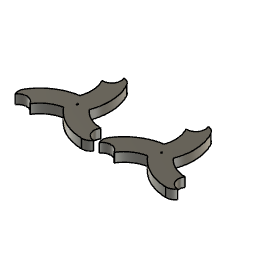
wheel v1 (Autodesk Fusion 360 design; units mm, degrees)
Autodesk Fusion 360 part; units mm, degrees
note: some values were not read from the file. Set by a fixed rule: which sketch regions a step uses.
sketch "스케치1" plane through (0, 0, 0) normal (0, 0, 1) x (1, 0, 0)
  arc A0 (-0.9923, 8.7365) -> (-0.9923, -1.7365) centre (2, 3.5) ccw
  arc A1 (0.9923, 5.2635) -> (-0.9923, 8.7365) centre (0, 7) ccw
  arc A2 (0.9923, 5.2635) -> (0.9923, 1.7365) centre (2, 3.5) ccw
  arc A3 (-0.9923, -1.7365) -> (0.9923, 1.7365) centre (0, 0) ccw
  arc A4 (0, 7) -> (0, 0) centre (2, 3.5) ccw construction
  arc A5 (-7.0699, -5.2276) -> (2, 0.0089) centre (-4.0311, -0.0179) ccw
  arc A6 (-5.0545, -1.7724) -> (-7.0699, -5.2276) centre (-6.0622, -3.5) ccw
  arc A7 (-6.0622, -3.5) -> (0, 0) centre (-4.0311, -0.0179) ccw construction
  arc A8 (-5.0545, -1.7724) -> (-2, -0.0089) centre (-4.0311, -0.0179) ccw
  arc A9 (2, 0.0089) -> (-2, -0.0089) centre (0, 0) ccw
  arc A10 (8.0622, -3.5089) -> (-1.0077, 1.7276) centre (2.0311, -3.4821) ccw
  arc A11 (4.0622, -3.4911) -> (8.0622, -3.5089) centre (6.0622, -3.5) ccw
  arc A12 (6.0622, -3.5) -> (0, 0) centre (2.0311, -3.4821) ccw construction
  arc A13 (4.0622, -3.4911) -> (1.0077, -1.7276) centre (2.0311, -3.4821) ccw
  arc A14 (-1.0077, 1.7276) -> (1.0077, -1.7276) centre (0, 0) ccw
  dimension "d7" = 4
  dimension "d9" = 360
  constraint tangent A0 A1
  constraint tangent A1 A2
  constraint tangent A2 A3
  constraint tangent A0 A3
  constraint coincident A3.centre A4.end
  measures "d7" diameter of A3
sketch "스케치2" plane through (0, 0, 0) normal (0, 0, 1) x (1, 0, 0)
  arc A0 (18.3127, 8.0738) -> (18.3127, -1.0738) centre (25.5, 3.5) ccw
  arc A1 (21.6873, 5.9262) -> (18.3127, 8.0738) centre (20, 7) ccw
  arc A2 (21.6873, 5.9262) -> (21.6873, 1.0738) centre (25.5, 3.5) ccw
  arc A3 (18.3127, -1.0738) -> (21.6873, 1.0738) centre (20, 0) ccw
  arc A4 (20, 7) -> (20, 0) centre (25.5, 3.5) ccw construction
  arc A5 (21.7736, -0.9244) -> (18.2264, 0.9244) centre (20, 0) ccw
  arc A6 (14.0241, -1.5019) -> (18.2264, 0.9244) centre (14.2189, 3.0131) ccw
  arc A7 (13.8516, -5.4981) -> (21.7736, -0.9244) centre (14.2189, 3.0131) ccw
  arc A8 (13.9378, -3.5) -> (20, 0) centre (14.2189, 3.0131) ccw construction
  arc A9 (14.0241, -1.5019) -> (13.8516, -5.4981) centre (13.9378, -3.5) ccw
  arc A10 (19.9138, 1.9981) -> (20.0862, -1.9981) centre (20, 0) ccw
  arc A11 (24.2886, -4.4244) -> (20.0862, -1.9981) centre (20.2811, -6.5131) ccw
  arc A12 (27.8357, -2.5756) -> (19.9138, 1.9981) centre (20.2811, -6.5131) ccw
  arc A13 (26.0622, -3.5) -> (20, 0) centre (20.2811, -6.5131) ccw construction
  arc A14 (24.2886, -4.4244) -> (27.8357, -2.5756) centre (26.0622, -3.5) ccw
  arc A15 (-21.3613, 8.4652) -> (-21.3613, -1.4652) centre (-16.7482, 3.5) ccw
  arc A16 (-18.6387, 5.5348) -> (-21.3613, 8.4652) centre (-20, 7) ccw
  arc A17 (-18.6387, 5.5348) -> (-18.6387, 1.4652) centre (-16.7482, 3.5) ccw
  arc A18 (-21.3613, -1.4652) -> (-18.6387, 1.4652) centre (-20, 0) ccw
  arc A19 (-20, 7) -> (-20, 0) centre (-16.7482, 3.5) ccw construction
  arc A20 (-18.0504, -0.4463) -> (-21.9496, 0.4463) centre (-20, 0) ccw
  arc A21 (-26.6504, -5.4115) -> (-18.0504, -0.4463) centre (-24.657, 1.0661) ccw
  arc A22 (-25.4739, -1.5885) -> (-26.6504, -5.4115) centre (-26.0622, -3.5) ccw
  arc A23 (-25.4739, -1.5885) -> (-21.9496, 0.4463) centre (-24.657, 1.0661) ccw
  arc A24 (-26.0622, -3.5) -> (-20, 0) centre (-24.657, 1.0661) ccw construction
  arc A25 (-20.5883, 1.9115) -> (-19.4117, -1.9115) centre (-20, 0) ccw
  arc A26 (-11.9883, -3.0537) -> (-20.5883, 1.9115) centre (-18.5948, -4.5661) ccw
  arc A27 (-15.8874, -3.9463) -> (-11.9883, -3.0537) centre (-13.9378, -3.5) ccw
  arc A28 (-15.8874, -3.9463) -> (-19.4117, -1.9115) centre (-18.5948, -4.5661) ccw
  arc A29 (-13.9378, -3.5) -> (-20, 0) centre (-18.5948, -4.5661) ccw construction
  dimension "d12" = 4
  dimension "d14" = 360
  dimension "d15" = 7
  dimension "d16" = 4
  dimension "d18" = 360
  constraint tangent A0 A1
  constraint tangent A1 A2
  constraint tangent A2 A3
  constraint tangent A0 A3
  constraint tangent A15 A16
  constraint tangent A16 A17
  constraint tangent A17 A18
  constraint tangent A15 A18
  measures "d12" diameter of A3
  measures "d15" distance of A18.centre A16.centre
  measures "d16" diameter of A18
sketch "스케치3" plane through (0, 0, 3) normal (0, 0, 1) x (-1, 0, 0)
  arc A0 (11.9883, 3.0537) -> (19.1945, -2.1847) centre (18.5948, 4.5661) ccw
  arc A1 (18.6387, -5.5348) -> (19.1945, -2.1847) centre (16.7482, -3.5) ccw
  arc A2 (18.6387, -5.5348) -> (21.3613, -8.4652) centre (20, -7) ccw
  arc A3 (21.3613, -8.4652) -> (22.2948, 0.3948) centre (16.7482, -3.5) ccw
  arc A4 (25.4739, 1.5885) -> (22.2948, 0.3948) centre (24.657, -1.0661) ccw
  arc A5 (25.4739, 1.5885) -> (26.6504, 5.4115) centre (26.0622, 3.5) ccw
  arc A6 (26.6504, 5.4115) -> (18.5107, 1.7899) centre (24.657, -1.0661) ccw
  arc A7 (15.8874, 3.9463) -> (18.5107, 1.7899) centre (18.5948, 4.5661) ccw
  arc A8 (15.8874, 3.9463) -> (11.9883, 3.0537) centre (13.9378, 3.5) ccw
  circle A9 centre (20, 0) radius 2.5
  arc A10 (-286.7011, -14.9378) -> (-286.7011, -55.0622) centre (-268.8401, -35) ccw
  arc A11 (-286.7011, -14.9378) -> (-313.2989, 14.9378) centre (-300, 0) ccw
  arc A12 (-313.2989, 14.9378) -> (-313.2989, -84.9378) centre (-268.8401, -35) ccw
  arc A13 (-313.2989, -84.9378) -> (-286.7011, -55.0622) centre (-300, -70) ccw
  arc A14 (-300, 0) -> (-300, -70) centre (-268.8401, -35) ccw construction
  arc A15 (-306.2871, -18.9861) -> (-219.7922, 30.9517) centre (-285.269, 44.4852) ccw
  arc A16 (-293.7129, 18.9861) -> (-258.9642, 39.0483) centre (-285.269, 44.4852) ccw
  arc A17 (-300, 0) -> (-239.3782, 35) centre (-285.269, 44.4852) ccw construction
  arc A18 (-219.7922, 30.9517) -> (-258.9642, 39.0483) centre (-239.3782, 35) ccw
  arc A19 (-293.7129, 18.9861) -> (-306.2871, -18.9861) centre (-300, 0) ccw
  arc A20 (-280.414, 4.0483) -> (-366.9089, 53.9861) centre (-345.8908, -9.4852) ccw
  arc A21 (-319.586, -4.0483) -> (-354.3347, 16.0139) centre (-345.8908, -9.4852) ccw
  arc A22 (-300, 0) -> (-360.6218, 35) centre (-345.8908, -9.4852) ccw construction
  arc A23 (-366.9089, 53.9861) -> (-354.3347, 16.0139) centre (-360.6218, 35) ccw
  arc A24 (-319.586, -4.0483) -> (-280.414, 4.0483) centre (-300, 0) ccw
  dimension "d21" = 5
  dimension "d22" = 70
  dimension "d23" = 40
  dimension "d25" = 360
  constraint tangent A10 A11
  constraint tangent A11 A12
  constraint tangent A12 A13
  constraint tangent A10 A13
  measures "d21" diameter of A9
  measures "d22" distance of A13.centre A11.centre
  measures "d23" diameter of A11
sketch "스케치4" plane through (0, 0, 33) normal (0, 0, 1) x (-1, 0, 0)
  arc A0 (-284.7746, 17.629) -> (-366.9089, 53.9861) centre (-345.8908, -9.4852) ccw
  arc A1 (-366.9089, 53.9861) -> (-354.3347, 16.0139) centre (-360.6218, 35) ccw
  arc A2 (-322.8798, 4.3711) -> (-354.3347, 16.0139) centre (-345.8908, -9.4852) ccw
  arc A3 (-322.8798, 4.3711) -> (-313.2989, -84.9378) centre (-268.8401, -35) ccw
  arc A4 (-313.2989, -84.9378) -> (-286.7011, -55.0622) centre (-300, -70) ccw
  arc A5 (-292.3456, -22) -> (-286.7011, -55.0622) centre (-268.8401, -35) ccw
  arc A6 (-292.3456, -22) -> (-219.7922, 30.9517) centre (-285.269, 44.4852) ccw
  arc A7 (-219.7922, 30.9517) -> (-258.9642, 39.0483) centre (-239.3782, 35) ccw
  arc A8 (-284.7746, 17.629) -> (-258.9642, 39.0483) centre (-285.269, 44.4852) ccw
  circle A9 centre (-300, 0) radius 2.5
  line L0 (-297.5, 0) -> (-302, 0)
  line L1 (-302, -1.5) -> (-302, 1.5)
  dimension "d28" = 5
  dimension "d29" = 4.5
  constraint coincident A9 L0.start
  constraint horizontal L0
  constraint coincident A9 L1.start
  constraint coincident A9 L1.end
  constraint perpendicular L0 L1
  measures "d28" diameter of A9
  measures "d29" distance of L0.start L0.end
sketch "스케치5" plane through (0, 0, 33) normal (0, 0, 1) x (-1, 0, 0)
  line L0 (-302, -1.5) -> (-302, 1.5)
  arc A0 (-297.5, 0) -> (-302, 1.5) centre (-300, 0) ccw
  arc A1 (-302, -1.5) -> (-297.5, 0) centre (-300, 0) ccw
  arc A2 (-284.7746, 17.629) -> (-366.9089, 53.9861) centre (-345.8908, -9.4852) ccw
  arc A3 (-366.9089, 53.9861) -> (-354.3347, 16.0139) centre (-360.6218, 35) ccw
  arc A4 (-322.8798, 4.3711) -> (-354.3347, 16.0139) centre (-345.8908, -9.4852) ccw
  arc A5 (-322.8798, 4.3711) -> (-313.2989, -84.9378) centre (-268.8401, -35) ccw
  arc A6 (-313.2989, -84.9378) -> (-286.7011, -55.0622) centre (-300, -70) ccw
  arc A7 (-292.3456, -22) -> (-286.7011, -55.0622) centre (-268.8401, -35) ccw
  arc A8 (-292.3456, -22) -> (-219.7922, 30.9517) centre (-285.269, 44.4852) ccw
  arc A9 (-219.7922, 30.9517) -> (-258.9642, 39.0483) centre (-239.3782, 35) ccw
  arc A10 (-284.7746, 17.629) -> (-258.9642, 39.0483) centre (-285.269, 44.4852) ccw
  arc A11 (-572, -21) -> (-572, -99) centre (-520, -60) ccw
  arc A12 (-572, -21) -> (-628, 21) centre (-600, 0) ccw
  arc A13 (-628, 21) -> (-628, -141) centre (-520, -60) ccw
  arc A14 (-628, -141) -> (-572, -99) centre (-600, -120) ccw
  arc A15 (-600, 0) -> (-600, -120) centre (-520, -60) ccw construction
  arc A16 (-604.1865, -34.7487) -> (-463.8904, 46.2513) centre (-588.0385, 99.282) ccw
  arc A17 (-463.8904, 46.2513) -> (-528.2635, 73.7487) centre (-496.077, 60) ccw
  arc A18 (-595.8135, 34.7487) -> (-604.1865, -34.7487) centre (-600, 0) ccw
  arc A19 (-595.8135, 34.7487) -> (-528.2635, 73.7487) centre (-588.0385, 99.282) ccw
  arc A20 (-600, 0) -> (-496.077, 60) centre (-588.0385, 99.282) ccw construction
  arc A21 (-567.8135, 13.7487) -> (-708.1096, 94.7487) centre (-691.9615, -39.282) ccw
  arc A22 (-708.1096, 94.7487) -> (-699.7365, 25.2513) centre (-703.923, 60) ccw
  arc A23 (-632.1865, -13.7487) -> (-567.8135, 13.7487) centre (-600, 0) ccw
  arc A24 (-632.1865, -13.7487) -> (-699.7365, 25.2513) centre (-691.9615, -39.282) ccw
  arc A25 (-600, 0) -> (-703.923, 60) centre (-691.9615, -39.282) ccw construction
  line L1 (-600.7031, -154.9929) -> (-600.7031, 95.0071)
  line L2 (-600.7031, 95.0071) -> (-395.9953, 127.228)
  arc A26 (398.7679, -18.3054) -> (398.7679, -101.6946) centre (452.9046, -60) ccw
  arc A27 (398.7679, -18.3054) -> (351.2321, 18.3054) centre (375, 0) ccw
  arc A28 (351.2321, 18.3054) -> (351.2321, -138.3054) centre (452.9046, -60) ccw
  arc A29 (351.2321, -138.3054) -> (398.7679, -101.6946) centre (375, -120) ccw
  arc A30 (375, 0) -> (375, -120) centre (452.9046, -60) ccw construction
  arc A31 (375, 0) -> (478.923, 60) centre (388.0092, 97.4673) ccw construction
  arc A32 (378.969, 29.7363) -> (371.031, -29.7363) centre (375, 0) ccw
  arc A33 (378.969, 29.7363) -> (451.1862, 71.4309) centre (388.0092, 97.4673) ccw
  arc A34 (371.031, -29.7363) -> (506.6599, 48.5691) centre (388.0092, 97.4673) ccw
  arc A35 (506.6599, 48.5691) -> (451.1862, 71.4309) centre (478.923, 60) ccw
  arc A36 (375, 0) -> (271.077, 60) centre (284.0862, -37.4673) ccw construction
  arc A37 (347.2631, -11.4309) -> (402.7369, 11.4309) centre (375, 0) ccw
  arc A38 (347.2631, -11.4309) -> (275.0459, 30.2637) centre (284.0862, -37.4673) ccw
  arc A39 (402.7369, 11.4309) -> (267.108, 89.7363) centre (284.0862, -37.4673) ccw
  arc A40 (267.108, 89.7363) -> (275.0459, 30.2637) centre (271.077, 60) ccw
  dimension "d33" = 70
  dimension "d35" = 360
  dimension "d36" = 250
  dimension "d37" = 60
  dimension "d39" = 360
  constraint tangent A11 A12
  constraint tangent A12 A13
  constraint tangent A13 A14
  constraint tangent A11 A14
  constraint coincident A14 L1.start
  constraint vertical L1
  constraint tangent A26 A27
  constraint tangent A27 A28
  constraint tangent A28 A29
  constraint tangent A26 A29
  measures "d33" diameter of A12
  measures "d36" distance of L1.start L1.end
  measures "d37" diameter of A27
extrude "돌출5" add sketch "스케치5" along normal blind 30 contours A26 A27 A33 A34 A35 A37 A39 | A27 A32 A37 | A26 A34 A37 | A26 A28 A29 A32 A34 A37 A38 | A27 A33 A39 | A27 A28 A32 A33 A38 A39 A40 | A28 A32 A38 makes body 1
sketch "스케치6" plane through (0, 0, 63) normal (0, 0, 1) x (-1, 0, 0)
  arc A0 (393.6401, 29.368) -> (267.108, 89.7363) centre (284.0862, -37.4673) ccw
  arc A1 (267.108, 89.7363) -> (275.0459, 30.2637) centre (271.077, 60) ccw
  arc A2 (340.2465, 1.4588) -> (275.0459, 30.2637) centre (284.0862, -37.4673) ccw
  arc A3 (340.2465, 1.4588) -> (351.2321, -138.3054) centre (452.9046, -60) ccw
  arc A4 (351.2321, -138.3054) -> (398.7679, -101.6946) centre (375, -120) ccw
  arc A5 (391.1134, -30.8268) -> (398.7679, -101.6946) centre (452.9046, -60) ccw
  arc A6 (391.1134, -30.8268) -> (506.6599, 48.5691) centre (388.0092, 97.4673) ccw
  arc A7 (506.6599, 48.5691) -> (451.1862, 71.4309) centre (478.923, 60) ccw
  arc A8 (393.6401, 29.368) -> (451.1862, 71.4309) centre (388.0092, 97.4673) ccw
  circle A9 centre (375, 0) radius 2.5
  line L0 (377.5, 0) -> (373, 0)
  line L1 (373, -1.5) -> (373, 1.5)
  dimension "d42" = 5
  constraint coincident A9 L0.start
  constraint horizontal L0
  constraint coincident A9 L1.start
  constraint coincident A9 L1.end
  constraint perpendicular L0 L1
  measures "d42" diameter of A9
extrude "돌출6" cut sketch "스케치6" against normal blind 30 contours A9 L0 L1 | A9 L0 L1 bodies 1
sketch "스케치7" plane through (0, 0, 0) normal (0, 0, 1) x (1, 0, 0)
  arc A0 (-151.4706, 14.1176) -> (-151.4706, 105.8824) centre (-237.5, 60) ccw
  arc A1 (-151.4706, 14.1176) -> (-98.5294, -14.1176) centre (-125, 0) ccw
  arc A2 (-98.5294, -14.1176) -> (-98.5294, 134.1176) centre (-237.5, 60) ccw
  arc A3 (-98.5294, 134.1176) -> (-151.4706, 105.8824) centre (-125, 120) ccw
  arc A4 (-125, 0) -> (-125, 120) centre (-237.5, 60) ccw construction
  circle A5 centre (-149.8217, 136.8488) radius 30
  arc A6 (-125, 0) -> (-228.923, -60) centre (-120.7115, -127.4279) ccw construction
  arc A7 (-123.9909, -29.983) -> (-126.0091, 29.983) centre (-125, 0) ccw
  circle A8 centre (-231.1037, -89.9206) radius 30
  arc A9 (-254.3846, -44.1346) -> (-203.4615, -75.8654) centre (-228.923, -60) ccw
  arc A10 (-126.0091, 29.983) -> (-254.3846, -44.1346) centre (-120.7115, -127.4279) ccw
  arc A11 (-123.9909, -29.983) -> (-203.4615, -75.8654) centre (-120.7115, -127.4279) ccw
  arc A12 (-125, 0) -> (-21.077, -60) centre (-16.7885, 67.4279) ccw construction
  arc A13 (-99.5385, 15.8654) -> (-150.4615, -15.8654) centre (-125, 0) ccw
  circle A14 centre (5.9254, -46.9281) radius 30
  arc A15 (-22.086, -89.983) -> (-20.0679, -30.017) centre (-21.077, -60) ccw
  arc A16 (-150.4615, -15.8654) -> (-22.086, -89.983) centre (-16.7885, 67.4279) ccw
  arc A17 (-99.5385, 15.8654) -> (-20.0679, -30.017) centre (-16.7885, 67.4279) ccw
  dimension "d45" = 120
  dimension "d46" = 60
  dimension "d47" = 60
  dimension "d49" = 360
  constraint tangent A0 A1
  constraint tangent A1 A2
  constraint tangent A2 A3
  constraint tangent A0 A3
  constraint coincident A3 A5.centre
  measures "d45" distance of A3.centre A1.centre
  measures "d46" diameter of A1
  measures "d47" diameter of A5
extrude "돌출7" add sketch "스케치7" along normal blind 30 separate body contours A0 A1 A8 A9 A10 A11 A13 A16 | A1 A7 A13 | A0 A10 A13 | A0 A2 A3 A5 A7 A10 A13 A17 | A1 A11 A16 | A1 A2 A7 A11 A14 A15 A16 A17 | A2 A7 A17 makes body 2
sketch "스케치8" plane through (0, 0, 30) normal (0, 0, 1) x (-1, 0, 0)
  arc A0 (18.8963, 30.0794) -> (20.0679, 30.017) centre (21.077, 60) ccw
  arc A1 (90.4592, -3.5618) -> (20.0679, 30.017) centre (16.7885, -67.4279) ccw
  arc A2 (90.4592, -3.5618) -> (98.5294, -134.1176) centre (237.5, -60) ccw
  arc A3 (98.5294, -134.1176) -> (122.8194, -149.9206) centre (125, -120) ccw
  arc A4 (152.0023, -106.9281) -> (122.8194, -149.9206) centre (149.8217, -136.8488) ccw
  arc A5 (152.0023, -106.9281) -> (151.4706, -105.8824) centre (125, -120) ccw
  arc A6 (145.355, -28.1323) -> (151.4706, -105.8824) centre (237.5, -60) ccw
  arc A7 (145.355, -28.1323) -> (254.3846, 44.1346) centre (120.7115, 127.4279) ccw
  arc A8 (254.3846, 44.1346) -> (255.9254, 73.0719) centre (228.923, 60) ccw
  arc A9 (204.1013, 76.8488) -> (255.9254, 73.0719) centre (231.1037, 89.9206) ccw
  arc A10 (204.1013, 76.8488) -> (203.4615, 75.8654) centre (228.923, 60) ccw
  arc A11 (139.1857, 31.6941) -> (203.4615, 75.8654) centre (120.7115, 127.4279) ccw
  arc A12 (139.1857, 31.6941) -> (22.086, 89.983) centre (16.7885, -67.4279) ccw
  arc A13 (22.086, 89.983) -> (-3.7448, 76.8488) centre (21.077, 60) ccw
  arc A14 (18.8963, 30.0794) -> (-3.7448, 76.8488) centre (-5.9254, 46.9281) ccw
  circle A15 centre (125, 0) radius 2.5
  line L0 (122.5, 0) -> (127, 0)
  line L1 (127, 1.5) -> (127, -1.5)
  dimension "d52" = 5
  dimension "d53" = 4.5
  constraint coincident A15 L0.start
  constraint horizontal L0
  constraint coincident A15 L1.start
  constraint coincident A15 L1.end
  constraint vertical L1
  measures "d52" diameter of A15
  measures "d53" distance of L0.start L0.end
extrude "돌출8" cut sketch "스케치8" against normal blind 30 contours A15 L0 L1 | A15 L0 L1 bodies 2
move_face "면 이동1" by (-8.1437, -1.2859, 0) 1 faces at (-396.6499, -0.5781, 63) on bodies 1
move_body "이동1" bodies 1 to x (1, 0, 0) y (0, 1, 0) z (0, 0, 1) at (-60, 0, 0)
sketch "스케치9" plane through (0, 0, 33) normal (0, 0, 1) x (-1, 0, 0)
copy_body "CopyPasteBodies1" bodies 2 makes body 3
move_body "이동2" bodies 3 to x (1, 0, 0) y (0, 1, 0) z (0, 0, 1) at (275, 0, 0)
hidden bodies 1
